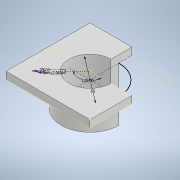
# Autodesk Inventor part: Parctica final.xx
Saved by Autodesk Inventor 2020 (Build 240168000, 168)
## iProperties
Created: 2020-04-21
Part Number: Parctica final.xx
Material: Genérico
Document SubType Name: Modeling
Designer: luisg
Density: 1 g/cm^3
Appearance: Valor por defecto
Author: luisg
Autodesk Inventor part; units mm, degrees
ref_plane "YZ Plane" through (0, 0, 0) normal (1, 0, 0) x (0, 1, 0)
ref_plane "XZ Plane" through (0, 0, 0) normal (0, 1, 0) x (-1, 0, 0)
ref_plane "XY Plane" through (0, 0, 0) normal (0, 0, 1) x (1, 0, 0)
sketch "Boceto1" plane through (0, 0, 0) normal (0, 1, 0) x (-1, 0, 0)
  line L0 (0, 0) -> (80, 0)
  line L1 (80, 0) -> (80, -80)
  line L2 (80, -80) -> (0, -80)
  line L3 (0, -80) -> (0, 0)
  dimension "d0" = 80
  dimension "d1" = 80
  constraints: 8 end point, 2 parallel, 1 horizontal, 1 perpendicular
  measures "d0" distance of L1.end L2.end
  measures "d1" distance of L0.end L1.end
extrude "Extrusión1" add sketch "Boceto1" along normal blind 7
sketch "Boceto2" plane through (0, 0, 0) normal (0, -1, 0) x (1, 0, 0)
  point P0 (0, 0)
sketch "Boceto3" plane through (0, 0, 0) normal (0, -1, 0) x (1, 0, 0)
  line L0 (-80, 0) -> (0, 0) construction
  line L1 (-40, 0) -> (-40, -80) construction
  line L2 (0, -80) -> (-80, -80) construction
  line L3 (-80, -80) -> (-80, 0) construction
  line L4 (-80, -40) -> (0, -40) construction
  line L5 (0, 0) -> (0, -80) construction
  circle A0 centre (-40, -40) radius 27.5
  dimension "d4" = 55
  constraints: 5 midpoint, 4 end point, 1 centre point
  measures "d4" diameter of A0
extrude "Extrusión2" add sketch "Boceto3" along normal blind 24
hole "Agujero1" at (-40, 0, -40) direction (0, 1, 0) diameter 40 end through all both
sketch "Boceto4" plane through (0, 7, 0) normal (0, 1, 0) x (1, 0, 0)
  circle A0 centre (-40, 40) radius 20 projected
  line L0 (-40, 40) -> (-40, 80)
  line L1 (0, 80) -> (-80, 80) projected
  line L2 (0, 80) -> (0, 40)
  line L3 (0, 0) -> (0, 80) projected
  line L4 (-40, 40) -> (0, 40)
  point P0 (-20, 40)
  point P1 (-40, 60)
  constraints: 6 end point, 2 midpoint, 1 perpendicular
extrude "Extrusión3" cut sketch "Boceto4" against normal through all contours A0 L0 L1 L2 L4
sketch "Boceto7" plane through (0, 7, 0) normal (0, 1, 0) x (1, 0, 0)
  line L0 (-40, 40) -> (-57.5963, 22.4037) construction
  line L1 (-80, 40) -> (0, 40) construction
  line L2 (-58.6139, 17.8506) -> (-50.0833, 26.3811)
  line L3 (-50.0833, 26.3811) -> (-53.6189, 29.9167)
  line L4 (-53.6189, 29.9167) -> (-62.1494, 21.3861)
  line L5 (-62.1494, 21.3861) -> (-58.6139, 17.8506)
  point P0 (0, 0)
  point P1 (-60.3816, 19.6184)
  dimension "d16" = 135
  dimension "d17" = 2.5
  dimension "d18" = 2.5
  dimension "d19" = 12.064
  constraints: 10 end point, 2 parallel, 1 perpendicular, 1 point on line
  measures "d16" angle of L1 L0
  measures "d17" distance of point (-60.382, 19.618) L2.start
  measures "d18" distance of point (-60.382, 19.618) L4.end
  measures "d19" distance of L2.start L2.end
sketch3d "Boceto 3D1"
